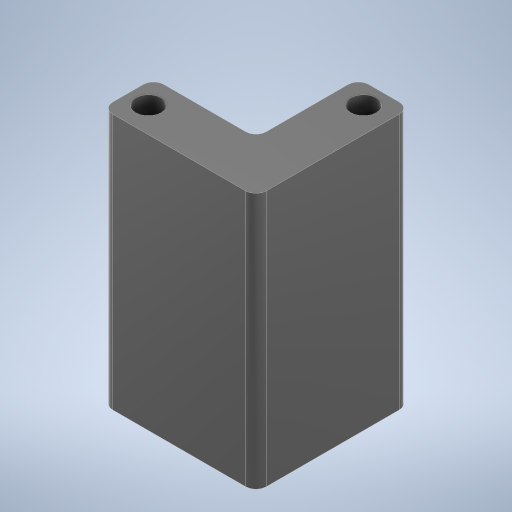
# Autodesk Inventor part: Base_3D Printed Beam
Saved by Autodesk Inventor 2024 (Build 280153000, 153)
## iProperties
Created: 2023-07-18
Part Number: Base_3D Printed Beam
Material: ABS Plastic
Document SubType Name: Modeling
Designer: javie
Density: 1.06 g/cm^3
Appearance: Sky Blue Medium
Author: javie
Autodesk Inventor part; units mm, degrees
ref_plane "YZ Plane" through (0, 0, 0) normal (1, 0, 0) x (0, 1, 0)
ref_plane "XZ Plane" through (0, 0, 0) normal (0, 1, 0) x (-1, 0, 0)
ref_plane "XY Plane" through (0, 0, 0) normal (0, 0, 1) x (1, 0, 0)
sketch "Sketch2" plane through (0, 0, 0) normal (0, 1, 0) x (-1, 0, 0)
  line L0 (-10, 10) -> (20, 10)
  line L1 (20, 10) -> (20, 0)
  line L2 (0, -20) -> (-10, -20)
  line L3 (-10, -20) -> (-10, 10)
  line L4 (0, 0) -> (20, 0)
  line L5 (20, 0) -> (20, -20)
  line L6 (20, -20) -> (0, -20)
  line L7 (0, -20) -> (0, 0)
  point P0 (5, 0)
  point P1 (0, -5)
  dimension "d4" = 30
  dimension "d5" = 30
  dimension "d6" = 20
  dimension "d7" = 20
  constraints: 16 end point, 4 parallel, 2 horizontal, 2 perpendicular, 1 coincident
  measures "d4" distance of L5.end L2.end
  measures "d5" distance of L0.end L5.end
  measures "d6" distance of L5.end L2.start
  measures "d7" distance of L5.end L1.end
extrude "Extrusion2" add sketch "Sketch2" along normal blind 50 contours L0 L1 L4 L7 L2 L3
sketch "Sketch3" plane through (0, 50, 0) normal (0, 1, 0) x (1, 0, 0)
  line L0 (10, 20) -> (0, 20) projected
  line L1 (0, 20) -> (0, 0) projected
  line L2 (-20, 0) -> (-20, -10) projected
  line L3 (-20, -10) -> (10, -10) projected
  point P0 (-16, -5)
  point P1 (5, 16)
  point P2 (-20, -5)
  point P3 (10, -10)
  point P4 (0, 5)
  dimension "d17" = 4
  dimension "d18" = 5
  dimension "d19" = 4
  dimension "d20" = 5
  constraints: 1 midpoint, 1 other
  measures "d17" distance from line of point (5, 16) L0
  measures "d18" distance from line of L1 point (5, 16)
  measures "d19" distance of point (-20, -5) point (-16, -5)
hole "Hole1" at (-16, 50, 5) at (5, 50, -16) direction (0, -1, 0) diameter 5 end through all
fillet "Fillet1" radius 2 2 edges at (10, 25, 10) (0, 25, 0)
fillet "Fillet2" radius 2 4 edges at (10, 25, -20) (0, 25, -20) (-20, 25, 0) (-20, 25, 10)
body "Solid2"
